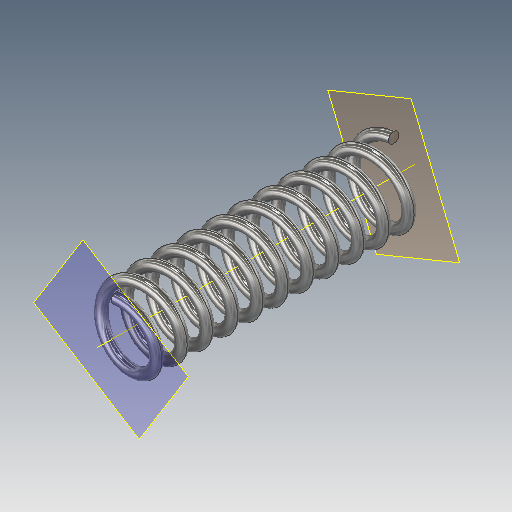
# Autodesk Inventor part: COIL SPRING
Saved by Autodesk Inventor 2019 (Build 230136000, 136)
## iProperties
Created: 2023-06-18
Part Number: COIL SPRING
Material: Generic
Document SubType Name: Modeling
Designer: Fransic
Density: 1 g/cm^3
Appearance: Chrome - Polished
Mass: 229.888 g
Surface Area: 840.824 cm^2
Volume: 229.888 cm^3
Author: Fransic
Autodesk Inventor part; units mm, degrees
ref_plane "YZ Plane" through (0, 0, 0) normal (1, 0, 0) x (0, 1, 0)
ref_plane "XZ Plane" through (0, 0, 0) normal (0, 1, 0) x (-1, 0, 0)
ref_plane "XY Plane" through (0, 0, 0) normal (0, 0, 1) x (1, 0, 0)
ref_plane "Work Plane1" through (0, -35.5, 290.7197) normal (0, 0, -1) x (-0.8488, 0.5287, 0)
ref_plane "Work Plane2" through (0, -35.5, -2.5303) normal (0, 0, 1) x (-0.3804, 0.9248, 0)
sketch "Sketch1" plane through (0, 0, 0) normal (1, 0, 0) x (0, 1, 0)
  line L0 (-8.2, -2.5303) -> (7.2, -2.5303) projected
  line L1 (7.2, 290.7197) -> (-8.2, 290.7197) projected
  circle A0 centre (-0.5, -2.5303) radius 5.5
  line L2 (-35.5, -10.2303) -> (-35.5, 5.1697) projected
  point P0 (0, 0)
  dimension "h0" = 293.25
  dimension "d1" = 11
  dimension "d2" = 35
  constraints: 1 centre point, 1 midpoint
  measures "h0" distance between parallel lines of L1 L0
  measures "d1" diameter of A0
  measures "d2" distance from line of L2 A0.centre
coil "Coil1" sketch "Sketch1" operation add axis through (0, -35.5, 0.7197) along (0, 0, 1) pitch 26.1591 turns 11 hand right
body "Solid1"
